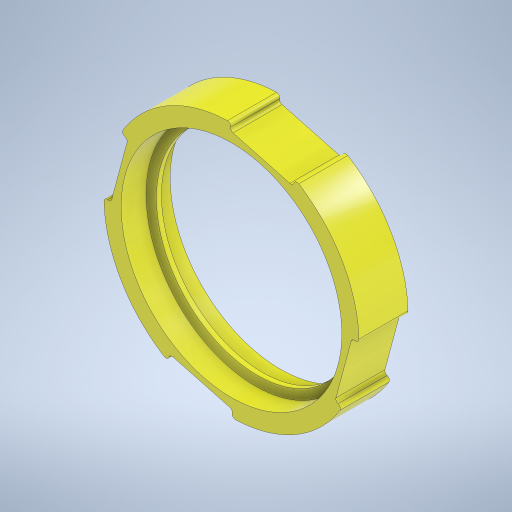
# Autodesk Inventor part: rosca_2
Saved by Autodesk Inventor 2023.2 (Build 272271030, 271C)
## iProperties
Created: 2023-10-23
Part Number: rosca_2
Material: Generic
Document SubType Name: Modeling
Designer: Cris Pat
Density: 1 g/cm^3
Appearance: Default
Author: Cris Pat
Autodesk Inventor part; units mm, degrees
ref_plane "YZ Plane" through (0, 0, 0) normal (1, 0, 0) x (0, 1, 0)
ref_plane "XZ Plane" through (0, 0, 0) normal (0, 1, 0) x (-1, 0, 0)
ref_plane "XY Plane" through (0, 0, 0) normal (0, 0, 1) x (1, 0, 0)
sketch "Sketch1" plane through (0, 0, 0) normal (0, 0, 1) x (1, 0, 0)
  circle A0 centre (0, 0) radius 31.2225
  dimension "d0" = 62.445
  constraints: 1 centre point, 1 coincident
  measures "d0" diameter of A0
extrude "Extrusion1" add sketch "Sketch1" against normal blind 12
sketch "Sketch2" plane through (0, 0, 0) normal (0, 0, 1) x (1, 0, 0)
  circle A0 centre (0, 0) radius 27
  dimension "d3" = 54
  constraints: 1 centre point, 1 coincident
  measures "d3" diameter of A0
extrude "Extrusion2" cut sketch "Sketch2" against normal through all
sketch "Sketch3" plane through (0, 0, 0) normal (1, 0, 0) x (0, 1, 0)
  line L0 (27, 0) -> (27, -12) construction
  line L1 (27, -12) -> (-27, -12) construction
  line L2 (27, -6.8664) -> (27, -9.1336)
  line L3 (27, -9.1336) -> (25, -8.6164)
  line L4 (25, -8.6164) -> (25, -7.3836)
  line L5 (25, -7.3836) -> (27, -6.8664)
  line L6 (-27, 0) -> (27, 0) construction
  point P0 (0, 0)
  point P1 (26, -8.875)
  point P2 (26, -7.125)
  point P3 (25, -8)
  dimension "d6" = 2
  dimension "d7" = 2
  dimension "d8" = 75.5
  dimension "d9" = 8
  constraints: 8 end point, 3 midpoint, 1 equal length, 1 parallel, 1 vertical, 1 vertical alignment
  measures "d6" distance between parallel lines of L4 L2
  measures "d8" angle of L3 L2
  measures "d9" distance from line of L6 point (25, -8)
coil "Coil1" sketch "Sketch3" operation add axis through (0, 0, -10) along (0, 0, 1) pitch 3 turns 1 hand right
chamfer "Chamfer1" distance 0.7 angle 45 4 edges at (0, 26, -4.125) (0, 26, -7.125) (0, 26, -5.875) (0, 26, -8.875)
sketch "Sketch4" plane through (0, 0, 0) normal (0, 0, 1) x (1, 0, 0)
  circle A0 centre (0, 0) radius 29.5 construction
  circle A1 centre (0, 0) radius 31.2225 construction
  line L0 (-0.3784, 29.4976) -> (15.0765, 25.3565)
  line L1 (15.0765, 25.3565) -> (15.8084, 28.0881)
  line L2 (15.8084, 28.0881) -> (0.3536, 32.2292)
  line L3 (0.3536, 32.2292) -> (-0.3784, 29.4976)
  line L4 (7.349, 27.427) -> (0, 0) construction
  line L5 (0, -44.8527) -> (0, 50.5586) construction
  point P0 (0, 31.2225)
  point P1 (15.4424, 26.7223)
  point P2 (-0.0124, 30.8634)
  dimension "d21" = 59
  dimension "d34" = 15
  dimension "d36" = 16
  constraints: 10 end point, 3 midpoint, 2 parallel, 2 point on circle, 1 centre point, 1 coincident, 1 perpendicular, 1 tangent, 1 vertical alignment
  measures "d21" diameter of A0
  measures "d34" angle of L4 L5
  measures "d36" distance of point (15.442, 26.722) point (-0.012, 30.863)
extrude "Extrusion3" cut sketch "Sketch4" against normal through all
fillet "Fillet1" radius 0.8 4 edges at (-0.3784, 29.4976, -6) (15.0765, 25.3565, -6) (0.0838, 31.2224, -6) (15.5386, 27.0813, -6)
pattern_circular "Circular Pattern1" count 4 over 360 about axis through (0, 0, -10) along (0, 0, 1) of "Fillet1", "Extrusion3"
sketch "Sketch5" plane through (0, 0, -12) normal (0, 0, -1) x (-1, 0, 0)
  arc A0 (6.3831, -27.6858) -> (8.315, -27.1682) centre (7.349, -27.427) ccw
  line L0 (8.315, -27.1682) -> (6.3831, -27.6858)
  line L1 (14.3037, -25.5635) -> (0.3944, -29.2905) construction
  point P0 (0, 0)
  dimension "d33" = 1
  constraints: 2 end point, 2 midpoint, 2 point on circle, 1 centre point, 1 coincident, 1 collinear
  measures "d33" radius of A0
extrude "Extrusion4" add sketch "Sketch5" against normal blind 5
fillet "Fillet2" radius 0.8 2 edges at (-6.3831, -27.6858, -9.5) (-8.315, -27.1682, -9.5)
body "Solid1"
